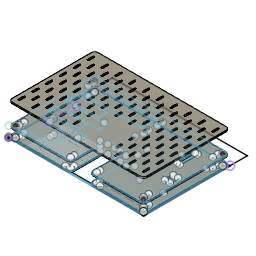
2025_09_22_ScreenToDK5 v7 (Autodesk Fusion 360 design; units mm, degrees)
Autodesk Fusion 360 part; units mm, degrees
(part 1 of 2)
sketch "WoodPlank" plane through (0, 0, 0) normal (0, 0, 1) x (1, 0, 0)
  line L0 (0, 0) -> (390, 0)
  line L1 (390, 0) -> (390, 300)
  line L2 (390, 300) -> (0, 300)
  line L3 (0, 300) -> (0, 0)
  line L4 (390, 0) -> (390, 10.3898)
  line L5 (390, 0) -> (390, 10.3898)
  line L6 (390, 0) -> (390, 250)
  line L7 (390, 250) -> (0, 250)
  line L8 (390, 0) -> (390, 5)
  line L9 (390, 5) -> (0, 5)
  line L10 (390, 0) -> (240, 0) construction
  line L11 (240, 0) -> (240, 20) construction
  line L12 (240, 20) -> (390, 20) construction
  line L13 (390, 20) -> (390, 0) construction
  dimension "d29" = 390
  dimension "d30" = 300
  dimension "d31" = 250
  dimension "d32" = 5
  dimension "d33" = 150
  dimension "d34" = 20
  constraint horizontal L0
  constraint vertical L1
  constraint horizontal L2
  constraint vertical L3
  constraint coincident L0.start L3.end
  constraint coincident L1 L4.end
  constraint perpendicular L0 L6
  constraint coincident L3 L7.end
  constraint perpendicular L3 L7
  constraint vertical L8
  constraint coincident L3 L9.end
  constraint perpendicular L3 L9
  constraint horizontal L10
  constraint vertical L11
  constraint horizontal L12
  constraint vertical L13
  measures "d29" distance of L0.start L0.end
  measures "d30" distance of L0.start L2.end
  measures "d31" distance of L0.end L6.end
  measures "d32" distance of L0.end L8.end
  measures "d33" distance of L0.end L10.end
  measures "d34" distance of L0.end L12.end
sketch "Skadis" plane through (0, 0, 0) normal (0, 0, 1) x (1, 0, 0)
  line L0 (-6.1628, 16.1319) -> (13.8372, 16.1319)
  line L1 (16.3372, 16.1319) -> (16.3372, 31.1319)
  arc A0 (16.3372, 31.1319) -> (11.3372, 31.1319) centre (13.8372, 31.1319) ccw
  line L2 (11.3372, 31.1319) -> (11.3372, 16.1319)
  arc A1 (11.3372, 16.1319) -> (16.3372, 16.1319) centre (13.8372, 16.1319) ccw
  line L3 (13.8372, 16.1319) -> (13.8372, 31.1319) construction
  line L4 (51.3372, 31.1319) -> (51.3372, 16.1319)
  arc A2 (51.3372, 16.1319) -> (56.3372, 16.1319) centre (53.8372, 16.1319) ccw
  line L5 (56.3372, 16.1319) -> (56.3372, 31.1319)
  arc A3 (56.3372, 31.1319) -> (51.3372, 31.1319) centre (53.8372, 31.1319) ccw
  line L6 (71.3372, 51.1319) -> (71.3372, 36.1319)
  arc A4 (71.3372, 36.1319) -> (76.3372, 36.1319) centre (73.8372, 36.1319) ccw
  line L7 (76.3372, 36.1319) -> (76.3372, 51.1319)
  arc A5 (76.3372, 51.1319) -> (71.3372, 51.1319) centre (73.8372, 51.1319) ccw
  line L8 (31.3372, 51.1319) -> (31.3372, 36.1319)
  arc A6 (31.3372, 36.1319) -> (36.3372, 36.1319) centre (33.8372, 36.1319) ccw
  arc A7 (36.3372, 51.1319) -> (31.3372, 51.1319) centre (33.8372, 51.1319) ccw
  line L9 (36.3372, 36.1319) -> (36.3372, 51.1319)
  arc A8 (96.3372, 31.1319) -> (91.3372, 31.1319) centre (93.8372, 31.1319) ccw
  arc A9 (111.3372, 36.1319) -> (116.3372, 36.1319) centre (113.8372, 36.1319) ccw
  arc A10 (156.3372, 51.1319) -> (151.3372, 51.1319) centre (153.8372, 51.1319) ccw
  arc A11 (91.3372, 16.1319) -> (96.3372, 16.1319) centre (93.8372, 16.1319) ccw
  line L10 (93.8372, 16.1319) -> (93.8372, 31.1319) construction
  line L11 (131.3372, 31.1319) -> (131.3372, 16.1319)
  line L12 (136.3372, 16.1319) -> (136.3372, 31.1319)
  arc A12 (136.3372, 31.1319) -> (131.3372, 31.1319) centre (133.8372, 31.1319) ccw
  line L13 (91.3372, 31.1319) -> (91.3372, 16.1319)
  line L14 (96.3372, 16.1319) -> (96.3372, 31.1319)
  arc A13 (131.3372, 16.1319) -> (136.3372, 16.1319) centre (133.8372, 16.1319) ccw
  line L15 (111.3372, 51.1319) -> (111.3372, 36.1319)
  line L16 (116.3372, 36.1319) -> (116.3372, 51.1319)
  arc A14 (151.3372, 36.1319) -> (156.3372, 36.1319) centre (153.8372, 36.1319) ccw
  line L17 (156.3372, 36.1319) -> (156.3372, 51.1319)
  line L18 (151.3372, 51.1319) -> (151.3372, 36.1319)
  arc A15 (116.3372, 51.1319) -> (111.3372, 51.1319) centre (113.8372, 51.1319) ccw
  arc A16 (271.3372, 36.1319) -> (276.3372, 36.1319) centre (273.8372, 36.1319) ccw
  arc A17 (316.3372, 51.1319) -> (311.3372, 51.1319) centre (313.8372, 51.1319) ccw
  line L19 (291.3372, 31.1319) -> (291.3372, 16.1319)
  line L20 (296.3372, 16.1319) -> (296.3372, 31.1319)
  arc A18 (296.3372, 31.1319) -> (291.3372, 31.1319) centre (293.8372, 31.1319) ccw
  arc A19 (291.3372, 16.1319) -> (296.3372, 16.1319) centre (293.8372, 16.1319) ccw
  line L21 (271.3372, 51.1319) -> (271.3372, 36.1319)
  line L22 (276.3372, 36.1319) -> (276.3372, 51.1319)
  arc A20 (311.3372, 36.1319) -> (316.3372, 36.1319) centre (313.8372, 36.1319) ccw
  line L23 (316.3372, 36.1319) -> (316.3372, 51.1319)
  line L24 (311.3372, 51.1319) -> (311.3372, 36.1319)
  arc A21 (276.3372, 51.1319) -> (271.3372, 51.1319) centre (273.8372, 51.1319) ccw
  arc A22 (336.3372, 31.1319) -> (331.3372, 31.1319) centre (333.8372, 31.1319) ccw
  arc A23 (351.3372, 36.1319) -> (356.3372, 36.1319) centre (353.8372, 36.1319) ccw
  arc A24 (331.3372, 16.1319) -> (336.3372, 16.1319) centre (333.8372, 16.1319) ccw
  line L25 (333.8372, 16.1319) -> (333.8372, 31.1319) construction
  line L26 (371.3372, 31.1319) -> (371.3372, 16.1319)
  line L27 (376.3372, 16.1319) -> (376.3372, 31.1319)
  arc A25 (376.3372, 31.1319) -> (371.3372, 31.1319) centre (373.8372, 31.1319) ccw
  line L28 (331.3372, 31.1319) -> (331.3372, 16.1319)
  line L29 (336.3372, 16.1319) -> (336.3372, 31.1319)
  arc A26 (371.3372, 16.1319) -> (376.3372, 16.1319) centre (373.8372, 16.1319) ccw
  line L30 (351.3372, 51.1319) -> (351.3372, 36.1319)
  line L31 (356.3372, 36.1319) -> (356.3372, 51.1319)
  arc A27 (356.3372, 51.1319) -> (351.3372, 51.1319) centre (353.8372, 51.1319) ccw
  arc A28 (16.3372, 71.1319) -> (11.3372, 71.1319) centre (13.8372, 71.1319) ccw
  arc A29 (31.3372, 76.1319) -> (36.3372, 76.1319) centre (33.8372, 76.1319) ccw
  arc A30 (76.3372, 91.1319) -> (71.3372, 91.1319) centre (73.8372, 91.1319) ccw
  arc A31 (11.3372, 56.1319) -> (16.3372, 56.1319) centre (13.8372, 56.1319) ccw
  line L32 (13.8372, 56.1319) -> (13.8372, 71.1319) construction
  line L33 (51.3372, 71.1319) -> (51.3372, 56.1319)
  line L34 (56.3372, 56.1319) -> (56.3372, 71.1319)
  arc A32 (56.3372, 71.1319) -> (51.3372, 71.1319) centre (53.8372, 71.1319) ccw
  line L35 (11.3372, 71.1319) -> (11.3372, 56.1319)
  line L36 (16.3372, 56.1319) -> (16.3372, 71.1319)
  arc A33 (51.3372, 56.1319) -> (56.3372, 56.1319) centre (53.8372, 56.1319) ccw
  line L37 (31.3372, 91.1319) -> (31.3372, 76.1319)
  line L38 (36.3372, 76.1319) -> (36.3372, 91.1319)
  arc A34 (71.3372, 76.1319) -> (76.3372, 76.1319) centre (73.8372, 76.1319) ccw
  line L39 (76.3372, 76.1319) -> (76.3372, 91.1319)
  line L40 (71.3372, 91.1319) -> (71.3372, 76.1319)
  arc A35 (36.3372, 91.1319) -> (31.3372, 91.1319) centre (33.8372, 91.1319) ccw
  arc A36 (96.3372, 71.1319) -> (91.3372, 71.1319) centre (93.8372, 71.1319) ccw
  arc A37 (111.3372, 76.1319) -> (116.3372, 76.1319) centre (113.8372, 76.1319) ccw
  arc A38 (156.3372, 91.1319) -> (151.3372, 91.1319) centre (153.8372, 91.1319) ccw
  arc A39 (91.3372, 56.1319) -> (96.3372, 56.1319) centre (93.8372, 56.1319) ccw
  line L41 (93.8372, 56.1319) -> (93.8372, 71.1319) construction
  line L42 (131.3372, 71.1319) -> (131.3372, 56.1319)
  line L43 (136.3372, 56.1319) -> (136.3372, 71.1319)
  arc A40 (136.3372, 71.1319) -> (131.3372, 71.1319) centre (133.8372, 71.1319) ccw
  line L44 (91.3372, 71.1319) -> (91.3372, 56.1319)
  line L45 (96.3372, 56.1319) -> (96.3372, 71.1319)
  arc A41 (131.3372, 56.1319) -> (136.3372, 56.1319) centre (133.8372, 56.1319) ccw
  line L46 (111.3372, 91.1319) -> (111.3372, 76.1319)
  line L47 (116.3372, 76.1319) -> (116.3372, 91.1319)
  arc A42 (151.3372, 76.1319) -> (156.3372, 76.1319) centre (153.8372, 76.1319) ccw
  line L48 (156.3372, 76.1319) -> (156.3372, 91.1319)
  line L49 (151.3372, 91.1319) -> (151.3372, 76.1319)
  arc A43 (116.3372, 91.1319) -> (111.3372, 91.1319) centre (113.8372, 91.1319) ccw
  arc A44 (271.3372, 76.1319) -> (276.3372, 76.1319) centre (273.8372, 76.1319) ccw
  arc A45 (316.3372, 91.1319) -> (311.3372, 91.1319) centre (313.8372, 91.1319) ccw
  line L50 (291.3372, 71.1319) -> (291.3372, 56.1319)
  line L51 (296.3372, 56.1319) -> (296.3372, 71.1319)
  arc A46 (296.3372, 71.1319) -> (291.3372, 71.1319) centre (293.8372, 71.1319) ccw
  arc A47 (291.3372, 56.1319) -> (296.3372, 56.1319) centre (293.8372, 56.1319) ccw
  line L52 (271.3372, 91.1319) -> (271.3372, 76.1319)
  line L53 (276.3372, 76.1319) -> (276.3372, 91.1319)
  arc A48 (311.3372, 76.1319) -> (316.3372, 76.1319) centre (313.8372, 76.1319) ccw
  line L54 (316.3372, 76.1319) -> (316.3372, 91.1319)
  line L55 (311.3372, 91.1319) -> (311.3372, 76.1319)
  arc A49 (276.3372, 91.1319) -> (271.3372, 91.1319) centre (273.8372, 91.1319) ccw
  arc A50 (336.3372, 71.1319) -> (331.3372, 71.1319) centre (333.8372, 71.1319) ccw
  arc A51 (351.3372, 76.1319) -> (356.3372, 76.1319) centre (353.8372, 76.1319) ccw
  arc A52 (331.3372, 56.1319) -> (336.3372, 56.1319) centre (333.8372, 56.1319) ccw
  line L56 (333.8372, 56.1319) -> (333.8372, 71.1319) construction
  line L57 (371.3372, 71.1319) -> (371.3372, 56.1319)
  line L58 (376.3372, 56.1319) -> (376.3372, 71.1319)
  arc A53 (376.3372, 71.1319) -> (371.3372, 71.1319) centre (373.8372, 71.1319) ccw
  line L59 (331.3372, 71.1319) -> (331.3372, 56.1319)
  line L60 (336.3372, 56.1319) -> (336.3372, 71.1319)
  arc A54 (371.3372, 56.1319) -> (376.3372, 56.1319) centre (373.8372, 56.1319) ccw
  line L61 (351.3372, 91.1319) -> (351.3372, 76.1319)
  line L62 (356.3372, 76.1319) -> (356.3372, 91.1319)
  arc A55 (356.3372, 91.1319) -> (351.3372, 91.1319) centre (353.8372, 91.1319) ccw
  arc A56 (16.3372, 111.1319) -> (11.3372, 111.1319) centre (13.8372, 111.1319) ccw
  arc A57 (31.3372, 116.1319) -> (36.3372, 116.1319) centre (33.8372, 116.1319) ccw
  arc A58 (76.3372, 131.1319) -> (71.3372, 131.1319) centre (73.8372, 131.1319) ccw
  arc A59 (11.3372, 96.1319) -> (16.3372, 96.1319) centre (13.8372, 96.1319) ccw
  line L63 (13.8372, 96.1319) -> (13.8372, 111.1319) construction
  line L64 (51.3372, 111.1319) -> (51.3372, 96.1319)
  line L65 (56.3372, 96.1319) -> (56.3372, 111.1319)
  arc A60 (56.3372, 111.1319) -> (51.3372, 111.1319) centre (53.8372, 111.1319) ccw
  line L66 (11.3372, 111.1319) -> (11.3372, 96.1319)
  line L67 (16.3372, 96.1319) -> (16.3372, 111.1319)
  arc A61 (51.3372, 96.1319) -> (56.3372, 96.1319) centre (53.8372, 96.1319) ccw
  line L68 (31.3372, 131.1319) -> (31.3372, 116.1319)
  line L69 (36.3372, 116.1319) -> (36.3372, 131.1319)
  arc A62 (71.3372, 116.1319) -> (76.3372, 116.1319) centre (73.8372, 116.1319) ccw
  line L70 (76.3372, 116.1319) -> (76.3372, 131.1319)
  line L71 (71.3372, 131.1319) -> (71.3372, 116.1319)
  arc A63 (36.3372, 131.1319) -> (31.3372, 131.1319) centre (33.8372, 131.1319) ccw
  arc A64 (96.3372, 111.1319) -> (91.3372, 111.1319) centre (93.8372, 111.1319) ccw
  arc A65 (111.3372, 116.1319) -> (116.3372, 116.1319) centre (113.8372, 116.1319) ccw
  arc A66 (156.3372, 131.1319) -> (151.3372, 131.1319) centre (153.8372, 131.1319) ccw
  arc A67 (91.3372, 96.1319) -> (96.3372, 96.1319) centre (93.8372, 96.1319) ccw
  line L72 (93.8372, 96.1319) -> (93.8372, 111.1319) construction
  line L73 (131.3372, 111.1319) -> (131.3372, 96.1319)
  line L74 (136.3372, 96.1319) -> (136.3372, 111.1319)
  arc A68 (136.3372, 111.1319) -> (131.3372, 111.1319) centre (133.8372, 111.1319) ccw
  line L75 (91.3372, 111.1319) -> (91.3372, 96.1319)
  line L76 (96.3372, 96.1319) -> (96.3372, 111.1319)
  arc A69 (131.3372, 96.1319) -> (136.3372, 96.1319) centre (133.8372, 96.1319) ccw
  line L77 (111.3372, 131.1319) -> (111.3372, 116.1319)
  line L78 (116.3372, 116.1319) -> (116.3372, 131.1319)
  arc A70 (151.3372, 116.1319) -> (156.3372, 116.1319) centre (153.8372, 116.1319) ccw
  line L79 (156.3372, 116.1319) -> (156.3372, 131.1319)
  line L80 (151.3372, 131.1319) -> (151.3372, 116.1319)
  arc A71 (116.3372, 131.1319) -> (111.3372, 131.1319) centre (113.8372, 131.1319) ccw
  arc A72 (191.3372, 116.1319) -> (196.3372, 116.1319) centre (193.8372, 116.1319) ccw
  arc A73 (236.3372, 131.1319) -> (231.3372, 131.1319) centre (233.8372, 131.1319) ccw
  line L81 (191.3372, 131.1319) -> (191.3372, 116.1319)
  line L82 (196.3372, 116.1319) -> (196.3372, 131.1319)
  arc A74 (231.3372, 116.1319) -> (236.3372, 116.1319) centre (233.8372, 116.1319) ccw
  line L83 (236.3372, 116.1319) -> (236.3372, 131.1319)
  line L84 (231.3372, 131.1319) -> (231.3372, 116.1319)
  arc A75 (196.3372, 131.1319) -> (191.3372, 131.1319) centre (193.8372, 131.1319) ccw
  arc A76 (271.3372, 116.1319) -> (276.3372, 116.1319) centre (273.8372, 116.1319) ccw
  arc A77 (316.3372, 131.1319) -> (311.3372, 131.1319) centre (313.8372, 131.1319) ccw
  line L85 (291.3372, 111.1319) -> (291.3372, 96.1319)
  line L86 (296.3372, 96.1319) -> (296.3372, 111.1319)
  arc A78 (296.3372, 111.1319) -> (291.3372, 111.1319) centre (293.8372, 111.1319) ccw
  arc A79 (291.3372, 96.1319) -> (296.3372, 96.1319) centre (293.8372, 96.1319) ccw
  line L87 (271.3372, 131.1319) -> (271.3372, 116.1319)
  line L88 (276.3372, 116.1319) -> (276.3372, 131.1319)
  arc A80 (311.3372, 116.1319) -> (316.3372, 116.1319) centre (313.8372, 116.1319) ccw
  line L89 (316.3372, 116.1319) -> (316.3372, 131.1319)
  line L90 (311.3372, 131.1319) -> (311.3372, 116.1319)
  arc A81 (276.3372, 131.1319) -> (271.3372, 131.1319) centre (273.8372, 131.1319) ccw
  arc A82 (336.3372, 111.1319) -> (331.3372, 111.1319) centre (333.8372, 111.1319) ccw
  arc A83 (351.3372, 116.1319) -> (356.3372, 116.1319) centre (353.8372, 116.1319) ccw
  arc A84 (331.3372, 96.1319) -> (336.3372, 96.1319) centre (333.8372, 96.1319) ccw
  line L91 (333.8372, 96.1319) -> (333.8372, 111.1319) construction
  line L92 (371.3372, 111.1319) -> (371.3372, 96.1319)
  line L93 (376.3372, 96.1319) -> (376.3372, 111.1319)
  arc A85 (376.3372, 111.1319) -> (371.3372, 111.1319) centre (373.8372, 111.1319) ccw
  line L94 (331.3372, 111.1319) -> (331.3372, 96.1319)
  line L95 (336.3372, 96.1319) -> (336.3372, 111.1319)
  arc A86 (371.3372, 96.1319) -> (376.3372, 96.1319) centre (373.8372, 96.1319) ccw
  line L96 (351.3372, 131.1319) -> (351.3372, 116.1319)
  line L97 (356.3372, 116.1319) -> (356.3372, 131.1319)
  arc A87 (356.3372, 131.1319) -> (351.3372, 131.1319) centre (353.8372, 131.1319) ccw
  arc A88 (16.3372, 151.1319) -> (11.3372, 151.1319) centre (13.8372, 151.1319) ccw
  arc A89 (31.3372, 156.1319) -> (36.3372, 156.1319) centre (33.8372, 156.1319) ccw
  arc A90 (76.3372, 171.1319) -> (71.3372, 171.1319) centre (73.8372, 171.1319) ccw
  arc A91 (11.3372, 136.1319) -> (16.3372, 136.1319) centre (13.8372, 136.1319) ccw
  line L98 (13.8372, 136.1319) -> (13.8372, 151.1319) construction
  line L99 (51.3372, 151.1319) -> (51.3372, 136.1319)
  line L100 (56.3372, 136.1319) -> (56.3372, 151.1319)
  arc A92 (56.3372, 151.1319) -> (51.3372, 151.1319) centre (53.8372, 151.1319) ccw
  line L101 (11.3372, 151.1319) -> (11.3372, 136.1319)
  line L102 (16.3372, 136.1319) -> (16.3372, 151.1319)
  arc A93 (51.3372, 136.1319) -> (56.3372, 136.1319) centre (53.8372, 136.1319) ccw
  line L103 (31.3372, 171.1319) -> (31.3372, 156.1319)
  line L104 (36.3372, 156.1319) -> (36.3372, 171.1319)
  arc A94 (71.3372, 156.1319) -> (76.3372, 156.1319) centre (73.8372, 156.1319) ccw
  line L105 (76.3372, 156.1319) -> (76.3372, 171.1319)
  line L106 (71.3372, 171.1319) -> (71.3372, 156.1319)
  arc A95 (36.3372, 171.1319) -> (31.3372, 171.1319) centre (33.8372, 171.1319) ccw
  arc A96 (96.3372, 151.1319) -> (91.3372, 151.1319) centre (93.8372, 151.1319) ccw
  arc A97 (111.3372, 156.1319) -> (116.3372, 156.1319) centre (113.8372, 156.1319) ccw
  arc A98 (156.3372, 171.1319) -> (151.3372, 171.1319) centre (153.8372, 171.1319) ccw
  arc A99 (91.3372, 136.1319) -> (96.3372, 136.1319) centre (93.8372, 136.1319) ccw
  line L107 (93.8372, 136.1319) -> (93.8372, 151.1319) construction
  line L108 (131.3372, 151.1319) -> (131.3372, 136.1319)
  line L109 (136.3372, 136.1319) -> (136.3372, 151.1319)
  arc A100 (136.3372, 151.1319) -> (131.3372, 151.1319) centre (133.8372, 151.1319) ccw
  line L110 (91.3372, 151.1319) -> (91.3372, 136.1319)
  line L111 (96.3372, 136.1319) -> (96.3372, 151.1319)
  arc A101 (131.3372, 136.1319) -> (136.3372, 136.1319) centre (133.8372, 136.1319) ccw
  line L112 (111.3372, 171.1319) -> (111.3372, 156.1319)
  line L113 (116.3372, 156.1319) -> (116.3372, 171.1319)
  arc A102 (151.3372, 156.1319) -> (156.3372, 156.1319) centre (153.8372, 156.1319) ccw
  line L114 (156.3372, 156.1319) -> (156.3372, 171.1319)
  line L115 (151.3372, 171.1319) -> (151.3372, 156.1319)
  arc A103 (116.3372, 171.1319) -> (111.3372, 171.1319) centre (113.8372, 171.1319) ccw
  arc A104 (176.3372, 151.1319) -> (171.3372, 151.1319) centre (173.8372, 151.1319) ccw
  arc A105 (191.3372, 156.1319) -> (196.3372, 156.1319) centre (193.8372, 156.1319) ccw
  arc A106 (236.3372, 171.1319) -> (231.3372, 171.1319) centre (233.8372, 171.1319) ccw
  arc A107 (171.3372, 136.1319) -> (176.3372, 136.1319) centre (173.8372, 136.1319) ccw
  line L116 (173.8372, 136.1319) -> (173.8372, 151.1319) construction
  line L117 (211.3372, 151.1319) -> (211.3372, 136.1319)
  line L118 (216.3372, 136.1319) -> (216.3372, 151.1319)
  arc A108 (216.3372, 151.1319) -> (211.3372, 151.1319) centre (213.8372, 151.1319) ccw
  line L119 (171.3372, 151.1319) -> (171.3372, 136.1319)
  line L120 (176.3372, 136.1319) -> (176.3372, 151.1319)
  arc A109 (211.3372, 136.1319) -> (216.3372, 136.1319) centre (213.8372, 136.1319) ccw
  line L121 (191.3372, 171.1319) -> (191.3372, 156.1319)
  line L122 (196.3372, 156.1319) -> (196.3372, 171.1319)
  arc A110 (231.3372, 156.1319) -> (236.3372, 156.1319) centre (233.8372, 156.1319) ccw
  line L123 (236.3372, 156.1319) -> (236.3372, 171.1319)
  line L124 (231.3372, 171.1319) -> (231.3372, 156.1319)
  arc A111 (196.3372, 171.1319) -> (191.3372, 171.1319) centre (193.8372, 171.1319) ccw
  arc A112 (256.3372, 151.1319) -> (251.3372, 151.1319) centre (253.8372, 151.1319) ccw
  arc A113 (271.3372, 156.1319) -> (276.3372, 156.1319) centre (273.8372, 156.1319) ccw
  arc A114 (316.3372, 171.1319) -> (311.3372, 171.1319) centre (313.8372, 171.1319) ccw
  arc A115 (251.3372, 136.1319) -> (256.3372, 136.1319) centre (253.8372, 136.1319) ccw
  line L125 (253.8372, 136.1319) -> (253.8372, 151.1319) construction
  line L126 (291.3372, 151.1319) -> (291.3372, 136.1319)
  line L127 (296.3372, 136.1319) -> (296.3372, 151.1319)
  arc A116 (296.3372, 151.1319) -> (291.3372, 151.1319) centre (293.8372, 151.1319) ccw
  line L128 (251.3372, 151.1319) -> (251.3372, 136.1319)
  line L129 (256.3372, 136.1319) -> (256.3372, 151.1319)
  arc A117 (291.3372, 136.1319) -> (296.3372, 136.1319) centre (293.8372, 136.1319) ccw
  line L130 (271.3372, 171.1319) -> (271.3372, 156.1319)
  line L131 (276.3372, 156.1319) -> (276.3372, 171.1319)
  arc A118 (311.3372, 156.1319) -> (316.3372, 156.1319) centre (313.8372, 156.1319) ccw
  line L132 (316.3372, 156.1319) -> (316.3372, 171.1319)
  line L133 (311.3372, 171.1319) -> (311.3372, 156.1319)
  arc A119 (276.3372, 171.1319) -> (271.3372, 171.1319) centre (273.8372, 171.1319) ccw
  arc A120 (336.3372, 151.1319) -> (331.3372, 151.1319) centre (333.8372, 151.1319) ccw
  arc A121 (351.3372, 156.1319) -> (356.3372, 156.1319) centre (353.8372, 156.1319) ccw
  arc A122 (331.3372, 136.1319) -> (336.3372, 136.1319) centre (333.8372, 136.1319) ccw
  line L134 (333.8372, 136.1319) -> (333.8372, 151.1319) construction
  line L135 (371.3372, 151.1319) -> (371.3372, 136.1319)
  line L136 (376.3372, 136.1319) -> (376.3372, 151.1319)
  arc A123 (376.3372, 151.1319) -> (371.3372, 151.1319) centre (373.8372, 151.1319) ccw
  line L137 (331.3372, 151.1319) -> (331.3372, 136.1319)
  line L138 (336.3372, 136.1319) -> (336.3372, 151.1319)
  arc A124 (371.3372, 136.1319) -> (376.3372, 136.1319) centre (373.8372, 136.1319) ccw
  line L139 (351.3372, 171.1319) -> (351.3372, 156.1319)
  line L140 (356.3372, 156.1319) -> (356.3372, 171.1319)
  arc A125 (356.3372, 171.1319) -> (351.3372, 171.1319) centre (353.8372, 171.1319) ccw
  arc A126 (16.3372, 191.1319) -> (11.3372, 191.1319) centre (13.8372, 191.1319) ccw
  arc A127 (31.3372, 196.1319) -> (36.3372, 196.1319) centre (33.8372, 196.1319) ccw
  arc A128 (76.3372, 211.1319) -> (71.3372, 211.1319) centre (73.8372, 211.1319) ccw
  arc A129 (11.3372, 176.1319) -> (16.3372, 176.1319) centre (13.8372, 176.1319) ccw
  line L141 (13.8372, 176.1319) -> (13.8372, 191.1319) construction
  line L142 (51.3372, 191.1319) -> (51.3372, 176.1319)
  line L143 (56.3372, 176.1319) -> (56.3372, 191.1319)
  arc A130 (56.3372, 191.1319) -> (51.3372, 191.1319) centre (53.8372, 191.1319) ccw
  line L144 (11.3372, 191.1319) -> (11.3372, 176.1319)
  line L145 (16.3372, 176.1319) -> (16.3372, 191.1319)
  arc A131 (51.3372, 176.1319) -> (56.3372, 176.1319) centre (53.8372, 176.1319) ccw
  line L146 (31.3372, 211.1319) -> (31.3372, 196.1319)
  line L147 (36.3372, 196.1319) -> (36.3372, 211.1319)
  arc A132 (71.3372, 196.1319) -> (76.3372, 196.1319) centre (73.8372, 196.1319) ccw
  line L148 (76.3372, 196.1319) -> (76.3372, 211.1319)
  line L149 (71.3372, 211.1319) -> (71.3372, 196.1319)
  arc A133 (36.3372, 211.1319) -> (31.3372, 211.1319) centre (33.8372, 211.1319) ccw
  arc A134 (96.3372, 191.1319) -> (91.3372, 191.1319) centre (93.8372, 191.1319) ccw
  arc A135 (111.3372, 196.1319) -> (116.3372, 196.1319) centre (113.8372, 196.1319) ccw
  arc A136 (156.3372, 211.1319) -> (151.3372, 211.1319) centre (153.8372, 211.1319) ccw
  arc A137 (91.3372, 176.1319) -> (96.3372, 176.1319) centre (93.8372, 176.1319) ccw
  line L150 (93.8372, 176.1319) -> (93.8372, 191.1319) construction
  line L151 (131.3372, 191.1319) -> (131.3372, 176.1319)
  line L152 (136.3372, 176.1319) -> (136.3372, 191.1319)
  arc A138 (136.3372, 191.1319) -> (131.3372, 191.1319) centre (133.8372, 191.1319) ccw
  line L153 (91.3372, 191.1319) -> (91.3372, 176.1319)
  line L154 (96.3372, 176.1319) -> (96.3372, 191.1319)
  arc A139 (131.3372, 176.1319) -> (136.3372, 176.1319) centre (133.8372, 176.1319) ccw
  line L155 (111.3372, 211.1319) -> (111.3372, 196.1319)
  line L156 (116.3372, 196.1319) -> (116.3372, 211.1319)
  arc A140 (151.3372, 196.1319) -> (156.3372, 196.1319) centre (153.8372, 196.1319) ccw
  line L157 (156.3372, 196.1319) -> (156.3372, 211.1319)
  line L158 (151.3372, 211.1319) -> (151.3372, 196.1319)
  arc A141 (116.3372, 211.1319) -> (111.3372, 211.1319) centre (113.8372, 211.1319) ccw
  arc A142 (176.3372, 191.1319) -> (171.3372, 191.1319) centre (173.8372, 191.1319) ccw
  arc A143 (191.3372, 196.1319) -> (196.3372, 196.1319) centre (193.8372, 196.1319) ccw
  arc A144 (236.3372, 211.1319) -> (231.3372, 211.1319) centre (233.8372, 211.1319) ccw
  arc A145 (171.3372, 176.1319) -> (176.3372, 176.1319) centre (173.8372, 176.1319) ccw
  line L159 (173.8372, 176.1319) -> (173.8372, 191.1319) construction
  line L160 (211.3372, 191.1319) -> (211.3372, 176.1319)
  line L161 (216.3372, 176.1319) -> (216.3372, 191.1319)
  arc A146 (216.3372, 191.1319) -> (211.3372, 191.1319) centre (213.8372, 191.1319) ccw
  line L162 (171.3372, 191.1319) -> (171.3372, 176.1319)
  line L163 (176.3372, 176.1319) -> (176.3372, 191.1319)
  arc A147 (211.3372, 176.1319) -> (216.3372, 176.1319) centre (213.8372, 176.1319) ccw
  line L164 (191.3372, 211.1319) -> (191.3372, 196.1319)
  line L165 (196.3372, 196.1319) -> (196.3372, 211.1319)
  arc A148 (231.3372, 196.1319) -> (236.3372, 196.1319) centre (233.8372, 196.1319) ccw
  line L166 (236.3372, 196.1319) -> (236.3372, 211.1319)
  line L167 (231.3372, 211.1319) -> (231.3372, 196.1319)
  arc A149 (196.3372, 211.1319) -> (191.3372, 211.1319) centre (193.8372, 211.1319) ccw
  arc A150 (256.3372, 191.1319) -> (251.3372, 191.1319) centre (253.8372, 191.1319) ccw
  arc A151 (271.3372, 196.1319) -> (276.3372, 196.1319) centre (273.8372, 196.1319) ccw
  arc A152 (316.3372, 211.1319) -> (311.3372, 211.1319) centre (313.8372, 211.1319) ccw
  arc A153 (251.3372, 176.1319) -> (256.3372, 176.1319) centre (253.8372, 176.1319) ccw
  line L168 (253.8372, 176.1319) -> (253.8372, 191.1319) construction
  line L169 (291.3372, 191.1319) -> (291.3372, 176.1319)
  line L170 (296.3372, 176.1319) -> (296.3372, 191.1319)
  arc A154 (296.3372, 191.1319) -> (291.3372, 191.1319) centre (293.8372, 191.1319) ccw
  line L171 (251.3372, 191.1319) -> (251.3372, 176.1319)
  line L172 (256.3372, 176.1319) -> (256.3372, 191.1319)
  arc A155 (291.3372, 176.1319) -> (296.3372, 176.1319) centre (293.8372, 176.1319) ccw
  line L173 (271.3372, 211.1319) -> (271.3372, 196.1319)
  line L174 (276.3372, 196.1319) -> (276.3372, 211.1319)
  arc A156 (311.3372, 196.1319) -> (316.3372, 196.1319) centre (313.8372, 196.1319) ccw
  line L175 (316.3372, 196.1319) -> (316.3372, 211.1319)
  line L176 (311.3372, 211.1319) -> (311.3372, 196.1319)
  arc A157 (276.3372, 211.1319) -> (271.3372, 211.1319) centre (273.8372, 211.1319) ccw
  arc A158 (336.3372, 191.1319) -> (331.3372, 191.1319) centre (333.8372, 191.1319) ccw
  arc A159 (351.3372, 196.1319) -> (356.3372, 196.1319) centre (353.8372, 196.1319) ccw
  arc A160 (331.3372, 176.1319) -> (336.3372, 176.1319) centre (333.8372, 176.1319) ccw
  line L177 (333.8372, 176.1319) -> (333.8372, 191.1319) construction
  line L178 (371.3372, 191.1319) -> (371.3372, 176.1319)
  line L179 (376.3372, 176.1319) -> (376.3372, 191.1319)
  arc A161 (376.3372, 191.1319) -> (371.3372, 191.1319) centre (373.8372, 191.1319) ccw
  line L180 (331.3372, 191.1319) -> (331.3372, 176.1319)
  line L181 (336.3372, 176.1319) -> (336.3372, 191.1319)
  arc A162 (371.3372, 176.1319) -> (376.3372, 176.1319) centre (373.8372, 176.1319) ccw
  line L182 (351.3372, 211.1319) -> (351.3372, 196.1319)
  line L183 (356.3372, 196.1319) -> (356.3372, 211.1319)
  arc A163 (356.3372, 211.1319) -> (351.3372, 211.1319) centre (353.8372, 211.1319) ccw
  arc A164 (16.3372, 231.1319) -> (11.3372, 231.1319) centre (13.8372, 231.1319) ccw
  arc A165 (11.3372, 216.1319) -> (16.3372, 216.1319) centre (13.8372, 216.1319) ccw
  line L184 (13.8372, 216.1319) -> (13.8372, 231.1319) construction
  line L185 (51.3372, 231.1319) -> (51.3372, 216.1319)
  line L186 (56.3372, 216.1319) -> (56.3372, 231.1319)
  arc A166 (56.3372, 231.1319) -> (51.3372, 231.1319) centre (53.8372, 231.1319) ccw
  line L187 (11.3372, 231.1319) -> (11.3372, 216.1319)
  line L188 (16.3372, 216.1319) -> (16.3372, 231.1319)
  arc A167 (51.3372, 216.1319) -> (56.3372, 216.1319) centre (53.8372, 216.1319) ccw
  arc A168 (96.3372, 231.1319) -> (91.3372, 231.1319) centre (93.8372, 231.1319) ccw
  arc A169 (91.3372, 216.1319) -> (96.3372, 216.1319) centre (93.8372, 216.1319) ccw
  line L189 (93.8372, 216.1319) -> (93.8372, 231.1319) construction
  line L190 (131.3372, 231.1319) -> (131.3372, 216.1319)
  line L191 (136.3372, 216.1319) -> (136.3372, 231.1319)
  arc A170 (136.3372, 231.1319) -> (131.3372, 231.1319) centre (133.8372, 231.1319) ccw
  line L192 (91.3372, 231.1319) -> (91.3372, 216.1319)
  line L193 (96.3372, 216.1319) -> (96.3372, 231.1319)
  arc A171 (131.3372, 216.1319) -> (136.3372, 216.1319) centre (133.8372, 216.1319) ccw
  arc A172 (176.3372, 231.1319) -> (171.3372, 231.1319) centre (173.8372, 231.1319) ccw
  arc A173 (171.3372, 216.1319) -> (176.3372, 216.1319) centre (173.8372, 216.1319) ccw
  line L194 (173.8372, 216.1319) -> (173.8372, 231.1319) construction
  line L195 (211.3372, 231.1319) -> (211.3372, 216.1319)
  line L196 (216.3372, 216.1319) -> (216.3372, 231.1319)
  arc A174 (216.3372, 231.1319) -> (211.3372, 231.1319) centre (213.8372, 231.1319) ccw
  line L197 (171.3372, 231.1319) -> (171.3372, 216.1319)
  line L198 (176.3372, 216.1319) -> (176.3372, 231.1319)
  arc A175 (211.3372, 216.1319) -> (216.3372, 216.1319) centre (213.8372, 216.1319) ccw
  arc A176 (256.3372, 231.1319) -> (251.3372, 231.1319) centre (253.8372, 231.1319) ccw
  arc A177 (251.3372, 216.1319) -> (256.3372, 216.1319) centre (253.8372, 216.1319) ccw
  line L199 (253.8372, 216.1319) -> (253.8372, 231.1319) construction
  line L200 (291.3372, 231.1319) -> (291.3372, 216.1319)
  line L201 (296.3372, 216.1319) -> (296.3372, 231.1319)
  arc A178 (296.3372, 231.1319) -> (291.3372, 231.1319) centre (293.8372, 231.1319) ccw
  line L202 (251.3372, 231.1319) -> (251.3372, 216.1319)
  line L203 (256.3372, 216.1319) -> (256.3372, 231.1319)
  arc A179 (291.3372, 216.1319) -> (296.3372, 216.1319) centre (293.8372, 216.1319) ccw
  arc A180 (336.3372, 231.1319) -> (331.3372, 231.1319) centre (333.8372, 231.1319) ccw
  arc A181 (331.3372, 216.1319) -> (336.3372, 216.1319) centre (333.8372, 216.1319) ccw
  line L204 (333.8372, 216.1319) -> (333.8372, 231.1319) construction
  line L205 (371.3372, 231.1319) -> (371.3372, 216.1319)
  line L206 (376.3372, 216.1319) -> (376.3372, 231.1319)
  arc A182 (376.3372, 231.1319) -> (371.3372, 231.1319) centre (373.8372, 231.1319) ccw
  line L207 (331.3372, 231.1319) -> (331.3372, 216.1319)
  line L208 (336.3372, 216.1319) -> (336.3372, 231.1319)
  arc A183 (371.3372, 216.1319) -> (376.3372, 216.1319) centre (373.8372, 216.1319) ccw
  point P0 (93.8372, 16.1319)
  point P1 (333.8372, 16.1319)
  point P2 (13.8372, 56.1319)
  point P3 (93.8372, 56.1319)
  point P4 (333.8372, 56.1319)
  point P5 (13.8372, 96.1319)
  point P6 (93.8372, 96.1319)
  point P7 (333.8372, 96.1319)
  point P8 (13.8372, 136.1319)
  point P9 (93.8372, 136.1319)
  point P10 (173.8372, 136.1319)
  point P11 (253.8372, 136.1319)
  point P12 (333.8372, 136.1319)
  point P13 (13.8372, 176.1319)
  point P14 (93.8372, 176.1319)
  point P15 (173.8372, 176.1319)
  point P16 (253.8372, 176.1319)
  point P17 (333.8372, 176.1319)
  point P18 (13.8372, 216.1319)
  point P19 (93.8372, 216.1319)
  point P20 (173.8372, 216.1319)
  point P21 (253.8372, 216.1319)
  point P22 (333.8372, 216.1319)
  dimension "d48" = 20
  dimension "d49" = 5
  dimension "d50" = 15
  dimension "d51" = 5
  dimension "d52" = 15
  dimension "d53" = 5
  dimension "d54" = 15
  dimension "d55" = 5
  dimension "d56" = 15
  dimension "d59" = 80
  dimension "d60" = 40
  constraint horizontal L0
  constraint tangent L1 A0
  constraint tangent A0 L2
  constraint parallel L1 L2
  constraint tangent L2 A1
  constraint tangent L1 A1
  constraint perpendicular L0 L3
  constraint coincident L0.end A1.centre
  constraint tangent L5 A3
  constraint tangent L4 A3
  constraint parallel L4 L5
  constraint tangent L4 A2
  constraint tangent A2 L5
  constraint tangent A7 L9
  constraint tangent L8 A7
  constraint parallel L8 L9
  constraint tangent L8 A6
  constraint tangent A6 L9
  constraint tangent L7 A5
  constraint tangent L6 A5
  constraint parallel L6 L7
  constraint tangent L6 A4
  constraint tangent A4 L7
  measures "d48" distance of L0.start L0.end
  measures "d49" diameter of A0
  measures "d50" distance of L0.end A0.centre
  measures "d51" diameter of A3
  measures "d52" distance of A2.centre A3.centre
  measures "d53" diameter of A7
  measures "d54" distance of A6.centre A7.centre
  measures "d55" diameter of A5
  measures "d56" distance of A4.centre A5.centre
sketch "ScreenHolder" plane through (0, 0, 0) normal (0, 0, 1) x (1, 0, 0)
  line L0 (169.1953, 94.937) -> (244.1953, 94.937) construction
  line L1 (244.1953, 94.937) -> (244.1953, 19.937) construction
  line L2 (244.1953, 19.937) -> (169.1953, 19.937) construction
  line L3 (169.1953, 19.937) -> (169.1953, 94.937) construction
  circle A0 centre (169.1953, 94.937) radius 1.55
  circle A1 centre (244.1953, 94.937) radius 1.55
  circle A2 centre (244.1953, 19.937) radius 1.55
  circle A3 centre (169.1953, 19.937) radius 1.55
  line L4 (256.6953, 107.437) -> (156.6953, 107.437) construction
  line L5 (156.6953, 107.437) -> (156.6953, 7.437) construction
  line L6 (156.6953, 7.437) -> (256.6953, 7.437) construction
  line L7 (256.6953, 7.437) -> (256.6953, 107.437) construction
  circle A4 centre (156.6953, 107.437) radius 3.15
  circle A5 centre (256.6953, 107.437) radius 3.15
  circle A6 centre (256.6953, 7.437) radius 3.15
  circle A7 centre (156.6953, 7.437) radius 3.15
  line L8 (170.2913, 93.8409) -> (154.4679, 109.6643) construction
  line L9 (169.1953, 37.8182) -> (156.6953, 31.2786) construction
  line L10 (256.6953, 7.437) -> (256.6953, -15.563) construction
  line L11 (156.6953, 107.437) -> (170.2913, 93.8409) construction
  line L12 (243.0993, 21.033) -> (256.6953, 7.437) construction
  line L13 (244.1953, 94.937) -> (243.0993, 93.8409) construction
  line L14 (170.2913, 21.033) -> (169.1953, 19.937) construction
  line L15 (256.6953, 107.437) -> (243.0993, 93.8409) construction
  line L16 (170.2913, 21.033) -> (156.6953, 7.437) construction
  line L17 (234.3705, 107.437) -> (179.0201, 107.437)
  line L18 (179.0201, 107.437) -> (179.0201, 7.437)
  line L19 (179.0201, 7.437) -> (234.3705, 7.437)
  line L20 (234.3705, 7.437) -> (234.3705, 107.437)
  line L21 (234.3705, 107.437) -> (179.0201, 7.437) construction
  line L22 (179.0201, 107.437) -> (234.3705, 7.437) construction
  line L23 (179.0201, 7.437) -> (234.3705, 7.437)
  line L24 (234.3705, 7.437) -> (234.3705, -50.7817)
  line L25 (234.3705, -50.7817) -> (179.0201, -50.7817)
  line L26 (179.0201, -50.7817) -> (179.0201, 7.437)
  circle A8 centre (256.6953, 7.437) radius 6.5
  circle A9 centre (156.6953, 7.437) radius 6.5
  line L27 (390, 0) -> (390, 10.3898)
  line L28 (259.8453, 7.437) -> (389.8453, 7.437)
  line L29 (156.0847, 10.5272) -> (31.0847, 10.5272) construction
  line L30 (31.0847, 10.5272) -> (31.0847, 14.3713) construction
  line L31 (31.0847, 14.3713) -> (31.0847, 39.3713) construction
  line L32 (31.0847, 39.3713) -> (-15.0758, 39.3713)
  line L33 (-15.0758, 39.3713) -> (-15.0758, 89.3713)
  line L34 (-15.0758, 89.3713) -> (31.0847, 89.3713)
  line L35 (31.0847, 89.3713) -> (31.0847, 39.3713)
  line L36 (31.0847, 89.3713) -> (80.5651, 89.3713)
  line L37 (80.5651, 89.3713) -> (80.5651, 39.3713)
  line L38 (80.5651, 39.3713) -> (31.0847, 39.3713)
  line L39 (31.0847, 39.3713) -> (31.0847, 89.3713)
  point P0 (206.6953, 57.437)
  dimension "d4" = 75
  dimension "d5" = 75
  dimension "d6" = 3.1
  dimension "d7" = 100
  dimension "d8" = 100
  dimension "d9" = 6.3
  dimension "d15" = 23
  dimension "d77" = 13
  dimension "d78" = 13
  dimension "d79" = 130
  dimension "d80" = 125
  dimension "d81" = 25
  dimension "d82" = 50
  constraint horizontal L0
  constraint vertical L1
  constraint horizontal L2
  constraint vertical L3
  constraint coincident L0.start L3.end
  constraint coincident L0.end L1.start
  constraint coincident L1.end L2.start
  constraint coincident L2.end L3.start
  constraint equal A0 A1
  constraint equal A0 A3
  constraint equal A0 A2
  constraint horizontal L4
  constraint perpendicular L4 L5
  constraint parallel L4 L6
  constraint parallel L5 L7
  constraint coincident L4.end L5.start
  constraint coincident L4.start L7.end
  constraint coincident L6.end L7.start
  constraint coincident L5.end L6.start
  constraint equal A4 A5
  constraint equal A4 A6
  constraint equal A4 A7
  constraint coincident A4 L8.end
  constraint coincident L5 L9.end
  constraint coincident L3 L9.start
  constraint coincident A0 L8.start
  constraint collinear L11 L12
  constraint coincident A2 L12.start
  constraint coincident A1 L13.end
  constraint collinear L13 L14
  constraint collinear L15 L16
  constraint coincident A3 L14.start
  constraint horizontal L17
  constraint perpendicular L17 L18
  constraint parallel L17 L19
  constraint parallel L18 L20
  constraint coincident L21 P0
  constraint coincident L22 P0
  constraint coincident L4 L17.start
  constraint horizontal L23
  constraint vertical L24
  constraint horizontal L25
  constraint vertical L26
  constraint concentric A6 A8
  constraint coincident A6 L28.start
  constraint perpendicular L27 L28
  constraint coincident A7 L29.start
  constraint perpendicular L5 L29
  constraint perpendicular L29 L30
  constraint perpendicular L29 L31
  constraint horizontal L32
  constraint vertical L33
  constraint horizontal L34
  constraint vertical L35
  constraint horizontal L36
  constraint vertical L37
  constraint horizontal L38
  constraint vertical L39
  measures "d4" distance of L0.start L0.end
  measures "d5" distance of L0.start L2.end
  measures "d6" diameter of A0
  measures "d7" distance of L5.end L6.end
  measures "d8" distance of L4.end L5.end
  measures "d9" diameter of A4
  measures "d15" distance of L6.end L10.end
  measures "d77" diameter of A8
  measures "d78" diameter of A9
  measures "d79" distance of L28.start L28.end
  measures "d80" distance of L29.start L29.end
  measures "d81" distance of L30.end L31.end
  measures "d82" distance of L31.end L34.end
sketch "RaspberryPiDevkKit" plane through (0, 0, 0) normal (0, 0, 1) x (1, 0, 0)
  line L0 (297.9103, 213.2433) -> (366.4103, 213.2433)
  line L1 (297.9103, 56.2433) -> (297.9103, 213.2433) construction
  line L2 (366.4103, 81.2433) -> (366.4103, 203.2433) construction
  line L3 (366.4103, 213.2433) -> (366.4103, 203.2433) construction
  line L4 (366.4103, 54.2433) -> (297.9103, 54.2433)
  circle A0 centre (297.9103, 203.2433) radius 0.85
  line L5 (297.9103, 81.2433) -> (366.4103, 81.2433) construction
  line L6 (380.4103, 56.2433) -> (366.4103, 56.2433)
  line L7 (297.9103, 203.2433) -> (297.9103, 213.2433) construction
  line L8 (297.9103, 213.2433) -> (288.9103, 213.2433)
  line L9 (297.9103, 81.2433) -> (366.4103, 81.2433) construction
  line L10 (297.9103, 203.2433) -> (297.9103, 81.2433) construction
  line L11 (366.4103, 203.2433) -> (297.9103, 203.2433) construction
  line L12 (366.4103, 213.2433) -> (380.4103, 213.2433)
  line L13 (288.9103, 56.2433) -> (297.9103, 56.2433)
  line L14 (366.4103, 81.2433) -> (366.4103, 54.2433) construction
  line L15 (366.4103, 203.2433) -> (297.9103, 203.2433) construction
  circle A1 centre (297.9103, 81.2433) radius 0.85
  line L16 (366.4103, 56.2433) -> (366.4103, 213.2433) construction
  line L17 (288.9103, 213.2433) -> (288.9103, 56.2433)
  line L18 (297.9103, 54.2433) -> (297.9103, 81.2433) construction
  circle A2 centre (366.4103, 81.2433) radius 0.85
  line L19 (380.4103, 213.2433) -> (380.4103, 56.2433)
  circle A3 centre (366.4103, 203.2433) radius 0.85
  line L20 (366.4103, 203.2433) -> (346.4103, 203.2433)
  line L21 (346.4103, 203.2433) -> (334.4103, 203.2433)
  line L22 (334.4103, 203.2433) -> (334.4103, 148.2433)
  line L23 (334.4103, 148.2433) -> (346.4103, 148.2433)
  line L24 (346.4103, 148.2433) -> (346.4103, 203.2433)
  line L25 (346.4103, 203.2433) -> (334.4103, 203.2433)
  line L26 (334.4103, 203.2433) -> (334.4103, 208.2433)
  line L27 (334.4103, 208.2433) -> (346.4103, 208.2433)
  line L28 (346.4103, 208.2433) -> (346.4103, 203.2433)
  line L29 (378.7342, 87.0489) -> (358.7342, 87.0489)
  line L30 (358.7342, 87.0489) -> (358.7342, 112.0489)
  line L31 (358.7342, 112.0489) -> (378.7342, 112.0489)
  line L32 (378.7342, 112.0489) -> (378.7342, 87.0489)
  point P0 (315.0523, 60.5375)
  dimension "d22" = 68.5
  dimension "d23" = 122
  dimension "d24" = 1.7
  dimension "d25" = 27
  dimension "d26" = 10
  dimension "d27" = 14
  dimension "d28" = 9
  dimension "d87" = 20
  dimension "d88" = 12
  dimension "d89" = 55
  dimension "d90" = 5
  dimension "d91" = 20
  dimension "d92" = 25
  constraint horizontal L5
  constraint vertical L2
  constraint horizontal L11
  constraint vertical L10
  constraint coincident A0.centre L7.start
  constraint coincident L2.end L3.end
  constraint coincident L2.start L5.end
  constraint coincident L5.start L9.start
  constraint equal A0 A3
  constraint equal A0 A2
  constraint equal A0 A1
  constraint horizontal L9
  constraint vertical L14
  constraint horizontal L4
  constraint vertical L18
  constraint horizontal L15
  constraint vertical L7
  constraint horizontal L0
  constraint vertical L3
  constraint horizontal L12
  constraint vertical L19
  constraint horizontal L6
  constraint vertical L16
  constraint horizontal L8
  constraint vertical L17
  constraint horizontal L13
  constraint vertical L1
  constraint perpendicular L3 L20
  constraint horizontal L21
  constraint vertical L22
  constraint horizontal L23
  constraint vertical L24
  constraint horizontal L25
  constraint vertical L26
  constraint horizontal L27
  constraint vertical L28
  constraint horizontal L29
  constraint vertical L30
  constraint horizontal L31
  constraint vertical L32
  measures "d22" distance of L2.start L5.start
  measures "d23" distance of A0.centre L5.start
  measures "d24" diameter of A0
  measures "d25" distance of L5.start L4.end
  measures "d26" distance of L2.end L0.end
  measures "d27" distance of L12.end L0.end
  measures "d28" distance of L8.end L0.start
  measures "d87" distance of L2.end L20.end
  measures "d88" distance of L20.end L21.end
  measures "d89" distance of L20.end L23.end
  measures "d90" distance of L20.end L27.end
  measures "d91" distance of L29.start L29.end
  measures "d92" distance of L29.start L31.end
sketch "ESP32" plane through (0, 0, 0) normal (0, 0, 1) x (1, 0, 0)
  line L0 (63.663, 96.6716) -> (63.663, 170.6716)
  line L1 (21.813, 173.4216) -> (21.813, 93.9216)
  line L2 (21.813, 93.9216) -> (105.513, 93.9216)
  line L3 (105.513, 93.9216) -> (105.513, 173.4216)
  line L4 (105.513, 173.4216) -> (21.813, 173.4216)
  line L5 (21.813, 93.9216) -> (21.813, 96.9216)
  line L6 (21.813, 96.9216) -> (24.813, 96.9216)
  line L7 (24.813, 96.9216) -> (24.813, 93.9216)
  line L8 (24.813, 93.9216) -> (21.813, 93.9216)
  line L9 (21.813, 173.4216) -> (21.813, 170.4216)
  line L10 (21.813, 170.4216) -> (24.813, 170.4216)
  line L11 (24.813, 170.4216) -> (24.813, 173.4216)
  line L12 (24.813, 173.4216) -> (21.813, 173.4216)
  line L13 (105.513, 173.4216) -> (105.513, 170.4216)
  line L14 (105.513, 170.4216) -> (102.513, 170.4216)
  line L15 (102.513, 170.4216) -> (102.513, 173.4216)
  line L16 (102.513, 173.4216) -> (105.513, 173.4216)
  line L17 (105.513, 93.9216) -> (105.513, 96.9216)
  line L18 (105.513, 96.9216) -> (102.513, 96.9216)
  line L19 (102.513, 96.9216) -> (102.513, 93.9216)
  line L20 (102.513, 93.9216) -> (105.513, 93.9216)
  circle A0 centre (23.313, 95.4216) radius 1.5
  circle A1 centre (23.313, 171.9216) radius 1.5
  circle A2 centre (104.013, 171.9216) radius 1.5
  circle A3 centre (104.013, 95.4216) radius 1.5
  line L21 (18.663, 176.1716) -> (18.663, 91.1716)
  line L22 (18.663, 91.1716) -> (108.663, 91.1716)
  line L23 (108.663, 91.1716) -> (108.663, 176.1716)
  line L24 (108.663, 176.1716) -> (18.663, 176.1716)
  line L25 (18.663, 176.1716) -> (108.663, 91.1716) construction
  line L26 (18.663, 91.1716) -> (108.663, 176.1716) construction
  point P0 (63.663, 133.6716)
  dimension "d35" = 74
  dimension "d36" = 79.5
  dimension "d37" = 83.7
  dimension "d38" = 3
  dimension "d39" = 3
  dimension "d40" = 3
  dimension "d41" = 3
  dimension "d42" = 3
  dimension "d43" = 3
  dimension "d44" = 3
  dimension "d45" = 3
  dimension "d46" = 85
  dimension "d47" = 90
  constraint perpendicular L1 L2
  constraint parallel L1 L3
  constraint parallel L2 L4
  constraint tangent L7 A0
  constraint tangent L11 A1
  constraint tangent L15 A2
  constraint tangent L19 A3
  constraint perpendicular L21 L22
  constraint parallel L21 L23
  constraint parallel L22 L24
  constraint coincident L25 P0
  constraint coincident L26 P0
  constraint midpoint L0 P0
  measures "d35" distance of L0.start L0.end
  measures "d36" distance of L2.end L3.end
  measures "d37" distance of L1.end L2.end
  measures "d38" distance of L1.end L5.end
  measures "d39" distance of L1.end L7.end
  measures "d40" distance of L1.start L9.end
  measures "d41" distance of L1.start L11.end
  measures "d42" distance of L3.end L13.end
  measures "d43" distance of L3.end L15.end
  measures "d44" distance of L2.end L17.end
  measures "d45" distance of L2.end L19.end
  measures "d46" distance of L22.end L23.end
  measures "d47" distance of L21.end L22.end
sketch "Arduino" plane through (0, 0, 0) normal (0, 0, 1) x (1, 0, 0)
  line L0 (168.1053, 174.147) -> (235.9425, 174.147)
  line L1 (235.9425, 174.147) -> (235.9425, 121.2591)
  line L2 (235.9425, 121.2591) -> (168.1053, 121.2591)
  line L3 (168.1053, 121.2591) -> (168.1053, 174.147)
  circle A0 centre (233.3588, 167.0532) radius 1.7385
  circle A1 centre (233.3588, 139.2014) radius 1.774
  circle A2 centre (183.1901, 123.803) radius 1.7744
  line L4 (233.3588, 139.2014) -> (183.1901, 139.2014) construction
  line L5 (183.1901, 139.2014) -> (183.1901, 123.803) construction
  line L6 (183.1901, 123.803) -> (233.3588, 123.803) construction
  line L7 (233.3588, 123.803) -> (233.3588, 139.2014) construction
  line L8 (233.3588, 167.0532) -> (183.1901, 167.0532) construction
  line L9 (183.1901, 167.0532) -> (183.1901, 182.4515) construction
  line L10 (183.1901, 182.4515) -> (233.3588, 182.4515) construction
  line L11 (233.3588, 182.4515) -> (233.3588, 167.0532) construction
  circle A3 centre (183.1901, 182.4515) radius 1.7744
  constraint horizontal L0
  constraint vertical L1
  constraint horizontal L2
  constraint vertical L3
  constraint horizontal L4
  constraint vertical L5
  constraint horizontal L6
  constraint vertical L7
  constraint coincident A2.centre L5.end
  constraint coincident A1.centre L4.start
  constraint horizontal L8
  constraint vertical L9
  constraint horizontal L10
  constraint vertical L11
  constraint coincident A0.centre L8.start
  constraint equal L5 L9
  constraint equal L4 L8
  constraint coincident L9.end L10.start
  constraint equal A2 A3
sketch "Sketch17" plane through (0, 0, 0) normal (0, 0, 1) x (1, 0, 0)
  line L0 (26.6957, 231.645) -> (196.6957, 231.645)
  line L1 (196.6957, 231.645) -> (196.6957, 186.645)
  line L2 (196.6957, 186.645) -> (26.6957, 186.645)
  line L3 (26.6957, 186.645) -> (26.6957, 231.645)
  dimension "d123" = 170
  dimension "d124" = 45
  measures "d123" distance of L0.start L0.end
  measures "d124" distance of L0.start L2.end
sketch "Sketch18" plane through (0, 0, 0) normal (0, 0, 1) x (1, 0, 0)
sketch "Sketch19" plane through (0, 0, 0) normal (0, 0, 1) x (1, 0, 0)
  line L0 (18.663, 174.9637) -> (110.0633, 174.9637)
  line L1 (110.0633, 174.9637) -> (110.0633, 151.1933)
  line L2 (110.0633, 151.1933) -> (18.663, 151.1933)
  line L3 (18.663, 151.1933) -> (18.663, 174.9637)
  line L4 (18.663, 115.8685) -> (110.0633, 115.8685)
  line L5 (110.0633, 115.8685) -> (110.0633, 93.6879)
  line L6 (110.0633, 93.6879) -> (18.663, 93.6879)
  line L7 (18.663, 93.6879) -> (18.663, 115.8685)
  line L8 (18.663, 176.1716) -> (18.663, 91.1716)
  constraint horizontal L0
  constraint vertical L1
  constraint horizontal L2
  constraint vertical L3
  constraint horizontal L4
  constraint vertical L5
  constraint horizontal L6
  constraint vertical L7
  constraint coincident L4.start L8
sketch "PlankTop" plane through (0, 0, 0) normal (0, 0, 1) x (1, 0, 0)
  line L0 (10, 0) -> (379.754, 0)
  line L1 (389.754, 10) -> (389.754, 238.8231)
  line L2 (379.754, 248.8231) -> (10, 248.8231)
  line L3 (0, 238.8231) -> (0, 10)
  arc A0 (10, 248.8231) -> (0, 238.8231) centre (10, 238.8231) ccw
  arc A1 (389.754, 238.8231) -> (379.754, 248.8231) centre (379.754, 238.8231) ccw
  arc A2 (379.754, 0) -> (389.754, 10) centre (379.754, 10) ccw
  arc A3 (0, 10) -> (10, 0) centre (10, 10) ccw
  circle A4 centre (10, 238.8231) radius 1.5
  circle A5 centre (379.754, 238.8231) radius 1.5
  circle A6 centre (379.754, 10) radius 1.5
  circle A7 centre (10, 10) radius 1.5
  point P0 (390, 250)
  dimension "d61" = 10
  dimension "d62" = 10
  dimension "d93" = 3
  dimension "d94" = 3
  dimension "d95" = 3
  dimension "d96" = 3
  constraint horizontal L0
  constraint vertical L1
  constraint horizontal L2
  constraint vertical L3
  constraint tangent L3 A0
  constraint tangent L2 A0
  constraint tangent L2 A1
  constraint tangent L1 A1
  constraint tangent L0 A2
  constraint tangent L1 A2
  constraint equal A1 A2
  constraint tangent L0 A3
  constraint tangent L3 A3
  constraint equal A1 A3
  constraint concentric A0 A4
  constraint concentric A1 A5
  constraint concentric A2 A6
  constraint concentric A3 A7
  measures "d61" radius of A0
  measures "d62" radius of A1
  measures "d93" diameter of A4
  measures "d94" diameter of A5
  measures "d95" diameter of A6
  measures "d96" diameter of A7
extrude "Extrude1" add sketch "WoodPlank" sketch "PlankTop" along normal blind 4 contours L1 L3 L4 L5 L6 L7 L9 of sketch 2 contours L0 L1 L2 L3 A0 A1 A2 A3 | A4 | A5 | A6 | A7 makes body 1
sketch "Sketch13" plane through (0, 0, 0) normal (0, 0, 1) x (1, 0, 0)
  circle A0 centre (379.754, 238.8231) radius 1.5
  circle A1 centre (10, 238.8231) radius 1.5
  circle A2 centre (10, 10) radius 1.5
  circle A3 centre (379.754, 10) radius 1.5
  point P0 (379.754, 238.8231)
  point P1 (10, 238.8231)
  point P2 (10, 10)
  point P3 (379.754, 10)
  dimension "d83" = 3
  dimension "d84" = 3
  dimension "d85" = 3
  dimension "d86" = 3
  constraint coincident P0 A0.centre
  constraint coincident P1 A1.centre
  constraint coincident P2 A2.centre
  constraint coincident P3 A3.centre
  measures "d83" diameter of A0
  measures "d84" diameter of A1
  measures "d85" diameter of A2
  measures "d86" diameter of A3
extrude "Extrude2" cut sketch "Arduino" along normal blind 30 contours A0 | A1 | A2 | A3 bodies 1
extrude "Extrude3" cut sketch "ESP32" along normal blind 15 contours A1 | A0 | A2 | A3 bodies 1
extrude "Extrude4" cut sketch "RaspberryPiDevkKit" along normal blind 20 contours A0 | A1 | A2 | A3 | L21 L22 L23 L24 L25 | L29 L30 L31 L32 bodies 1